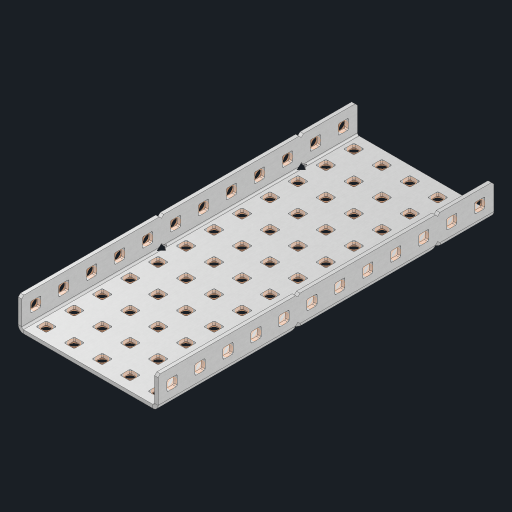
# Autodesk Inventor part: Alu C 1x3x1x35
Saved by Autodesk Inventor 2023 (Build 270158000, 158)
## iProperties
Created: 2022-07-28
Part Number: Alu C 1x3x1x35
Material: Generic
Document SubType Name: Sheet Metal
Designer: ylu12
Density: 1 g/cm^3
Sheet Metal Rule: Default
Appearance: VEX Alu
Author: ylu12
Autodesk Inventor part; units mm, degrees
ref_plane "YZ Plane" through (0, 0, 0) normal (1, 0, 0) x (0, 1, 0)
ref_plane "XZ Plane" through (0, 0, 0) normal (0, 1, 0) x (-1, 0, 0)
sketch "Sketch1" plane through (0, 0, 0) normal (0, 1, 0) x (-1, 0, 0)
  line L0 (-31.75, 0) -> (31.75, 0)
  line L1 (31.75, 0) -> (31.75, -152.4)
  line L2 (31.75, -152.4) -> (-31.75, -152.4)
  line L3 (-31.75, -152.4) -> (-31.75, 0)
  line L4 (31.75, 0) -> (-31.75, -152.4) construction
  point P0 (0, 0)
  point P1 (0, 0)
  dimension "d0" = 63.5
  dimension "d1" = 152.4
  measures "d0" distance of L1.end L2.end
  measures "d1" distance of L0.end L1.end
extrude "Plate1" add sketch "Sketch1" along normal blind 1.5875
sketch "Sketch2" plane through (30.1625, 0, -152.4) normal (1, 0, 0) x (0, 1, 0)
  line L0 (0, 152.4) -> (0, 0)
  line L1 (0, 0) -> (14.2875, 0)
  line L2 (14.2875, 0) -> (14.2875, 152.4)
  line L3 (14.2875, 152.4) -> (0, 152.4)
  constraints: 6 end point, 1 horizontal, 1 perpendicular, 1 vertical
edge flange "Flanges" height 12.7 angle 90 thickness 1.5875 bend radius 0.7937 thickness toward (1, 0, 0) relief tear relief width 1.5875 relief depth 0.7937 corner gap 1.5875 corner form 0 edges at (31.75, 1.5875, -76.2) (-31.75, 1.5875, -76.2) wall of the first edge with corners at (30.1625, 0, 0) (30.1625, 0, -152.4) (30.1625, 14.2875, -152.4) (30.1625, 14.2875, 0)
bend "Bend1"
corner "Corner1"
sketch "Sketch3" plane through (31.75, 2.3813, -152.4) normal (1, 0, 0) x (0, 0, -1)
  line L0 (-147.8534, 7.8676) -> (-144.2466, 7.8676)
  line L1 (-143.7386, 7.3597) -> (-143.7386, 3.7528)
  line L2 (-144.2466, 3.2448) -> (-147.8534, 3.2448)
  line L3 (-148.3614, 3.7528) -> (-148.3614, 7.3597)
  arc A0 (-147.8534, 7.8676) -> (-148.3614, 7.3597) centre (-147.8534, 7.3596) ccw
  arc A1 (-143.7386, 7.3597) -> (-144.2466, 7.8676) centre (-144.2466, 7.3596) ccw
  arc A2 (-144.2466, 3.2448) -> (-143.7386, 3.7528) centre (-144.2466, 3.7528) ccw
  arc A3 (-148.3614, 3.7528) -> (-147.8534, 3.2448) centre (-147.8534, 3.7528) ccw
  line L4 (-152.4, 0) -> (-152.4, 11.9062) construction
  line L5 (-152.4, 11.9062) -> (0, 11.9062) construction
  line L6 (-147.8534, 7.3596) -> (-144.2466, 3.7528) construction
  point P0 (-152.4, -2.3813)
  point P1 (-143.7386, 3.2448)
  point P2 (-148.3614, 3.2448)
  point P3 (-146.05, 5.5562)
  dimension "d16" = 4.6228
  dimension "d17" = 0.508
  dimension "d20" = 6.35
  dimension "d21" = 6.35
  constraints: 10 end point, 8 point on circle, 8 tangent, 4 centre point, 4 point on line, 3 equal radius, 2 parallel, 2 perpendicular, 1 horizontal, 1 midpoint
  measures "d16" distance of point (-143.739, 3.245) point (-148.361, 3.245)
  measures "d17" radius of A0
  measures "d20" distance from line of point (-146.05, 5.556) L4
  measures "d21" distance from line of L5 point (-146.05, 5.556)
extrude "Flange Stamp" cut sketch "Sketch3" against normal blind 1.5875
sketch "Sketch7" plane through (31.75, 2.3813, 0) normal (1, 0, 0) x (0, 0, -1)
  arc A0 (4.5466, 7.8677) -> (4.0386, 7.3597) centre (4.5466, 7.3597) ccw construction
  arc A1 (8.1534, 3.2449) -> (8.6614, 3.7529) centre (8.1534, 3.7529) ccw construction
  circle A2 centre (6.35, 5.5563) radius 2.1844
  line L0 (4.5466, 7.3597) -> (8.1534, 3.7529) construction
  point P0 (0, -2.3812)
  dimension "d46" = 4.3688
  constraints: 2 end point, 1 centre point, 1 midpoint
  measures "d46" diameter of A2
surface extrude "Flange Circle" sketch "Sketch7" against normal up to surface (1.5875 mm away) shown yes curves A2
ref_plane "Flange Pattern Plane" through (31.75, 7.9375, -4.5466) normal (0, 1, 0) x (1, 0, 0)
pattern_sketch "Flange Pattern" of "Flange Circle", "Flange Stamp" from (31.75, 7.9375, -6.35) facing (1, 0, 0) copies at (31.75, 7.9375, -19.05) facing (1, 0, 0) at (31.75, 7.9375, -31.75) facing (1, 0, 0) at (31.75, 7.9375, -44.45) facing (1, 0, 0) at (31.75, 7.9375, -57.15) facing (1, 0, 0) at (31.75, 7.9375, -69.85) facing (1, 0, 0) at (31.75, 7.9375, -82.55) facing (1, 0, 0) at (31.75, 7.9375, -95.25) facing (1, 0, 0) at (31.75, 7.9375, -107.95) facing (1, 0, 0) at (31.75, 7.9375, -120.65) facing (1, 0, 0) at (31.75, 7.9375, -133.35) facing (1, 0, 0) at (31.75, 7.9375, -146.05) facing (1, 0, 0) at (-31.75, 7.9375, -6.35) facing (-1, 0, 0) at (-31.75, 7.9375, -19.05) facing (-1, 0, 0) at (-31.75, 7.9375, -31.75) facing (-1, 0, 0) at (-31.75, 7.9375, -44.45) facing (-1, 0, 0) at (-31.75, 7.9375, -57.15) facing (-1, 0, 0) at (-31.75, 7.9375, -69.85) facing (-1, 0, 0) at (-31.75, 7.9375, -82.55) facing (-1, 0, 0) at (-31.75, 7.9375, -95.25) facing (-1, 0, 0) at (-31.75, 7.9375, -107.95) facing (-1, 0, 0) at (-31.75, 7.9375, -120.65) facing (-1, 0, 0) at (-31.75, 7.9375, -133.35) facing (-1, 0, 0) at (-31.75, 7.9375, -146.05) facing (-1, 0, 0)
sketch "Sketch8" plane through (0, 0, 0) normal (0, -1, 0) x (1, 0, 0)
  line L0 (29.3687, 0) -> (-29.3687, 0) construction
  line L1 (27.2034, -4.0386) -> (23.5966, -4.0386)
  line L2 (23.0886, -4.5466) -> (23.0886, -8.1534)
  line L3 (23.5966, -8.6614) -> (27.2034, -8.6614)
  line L4 (27.7114, -8.1534) -> (27.7114, -4.5466)
  arc A0 (27.7114, -4.5466) -> (27.2034, -4.0386) centre (27.2034, -4.5466) ccw
  arc A1 (27.2034, -8.6614) -> (27.7114, -8.1534) centre (27.2034, -8.1534) ccw
  arc A2 (23.0886, -8.1534) -> (23.5966, -8.6614) centre (23.5966, -8.1534) ccw
  arc A3 (23.5966, -4.0386) -> (23.0886, -4.5466) centre (23.5966, -4.5466) ccw
  line L5 (27.2034, -4.5466) -> (23.5966, -8.1534) construction
  line L6 (31.75, 0) -> (31.75, -152.4) construction
  point P0 (0, 0)
  point P1 (23.0886, -8.6614)
  point P2 (27.7114, -8.6614)
  point P3 (25.4, -6.35)
  dimension "d49" = 4.6228
  dimension "d50" = 0.508
  dimension "d51" = 6.35
  dimension "d52" = 6.35
  constraints: 10 end point, 8 point on circle, 8 tangent, 4 centre point, 4 point on line, 3 equal radius, 2 parallel, 2 perpendicular, 1 horizontal, 1 midpoint
  measures "d49" distance of point (27.711, -8.661) point (23.089, -8.661)
  measures "d50" radius of A0
  measures "d51" distance from line of L6 point (25.4, -6.35)
  measures "d52" distance from line of L0 point (25.4, -6.35)
extrude "Body Stamp" cut sketch "Sketch8" against normal blind 1.5875
sketch "Sketch9" plane through (0, 0, 0) normal (0, -1, 0) x (1, 0, 0)
  arc A0 (27.7114, -4.5466) -> (27.2034, -4.0386) centre (27.2034, -4.5466) ccw construction
  arc A1 (23.0886, -8.1534) -> (23.5966, -8.6614) centre (23.5966, -8.1534) ccw construction
  line L0 (27.2034, -4.5466) -> (23.5966, -8.1534) construction
  circle A2 centre (25.4, -6.35) radius 2.1844
  point P0 (0, 0)
  dimension "d55" = 4.3688
  constraints: 2 end point, 1 centre point, 1 midpoint
  measures "d55" diameter of A2
surface extrude "Body Circle" sketch "Sketch9" against normal up to surface (1.5875 mm away) shown yes curves A2
pattern_sketch "Body Pattern" of "Body Stamp", "Body Circle" from (25.4, 0, -6.35) copies at (25.4, 0, -19.05) at (25.4, 0, -31.75) at (25.4, 0, -44.45) at (25.4, 0, -57.15) at (25.4, 0, -69.85) at (25.4, 0, -82.55) at (25.4, 0, -95.25) at (25.4, 0, -107.95) at (25.4, 0, -120.65) at (25.4, 0, -133.35) at (25.4, 0, -146.05) at (12.7, 0, -6.35) at (12.7, 0, -19.05) at (12.7, 0, -31.75) at (12.7, 0, -44.45) at (12.7, 0, -57.15) at (12.7, 0, -69.85) at (12.7, 0, -82.55) at (12.7, 0, -95.25) at (12.7, 0, -107.95) at (12.7, 0, -120.65) at (12.7, 0, -133.35) at (12.7, 0, -146.05) at (0, 0, -6.35) at (0, 0, -19.05) at (0, 0, -31.75) at (0, 0, -44.45) at (0, 0, -57.15) at (0, 0, -69.85) at (0, 0, -82.55) at (0, 0, -95.25) at (0, 0, -107.95) at (0, 0, -120.65) at (0, 0, -133.35) at (0, 0, -146.05) at (-12.7, 0, -6.35) at (-12.7, 0, -19.05) at (-12.7, 0, -31.75) at (-12.7, 0, -44.45) at (-12.7, 0, -57.15) at (-12.7, 0, -69.85) at (-12.7, 0, -82.55) at (-12.7, 0, -95.25) at (-12.7, 0, -107.95) at (-12.7, 0, -120.65) at (-12.7, 0, -133.35) at (-12.7, 0, -146.05) at (-25.4, 0, -6.35) at (-25.4, 0, -19.05) at (-25.4, 0, -31.75) at (-25.4, 0, -44.45) at (-25.4, 0, -57.15) at (-25.4, 0, -69.85) at (-25.4, 0, -82.55) at (-25.4, 0, -95.25) at (-25.4, 0, -107.95) at (-25.4, 0, -120.65) at (-25.4, 0, -133.35) at (-25.4, 0, -146.05)
sketch "Arc Length" plane through (30.1625, 2.3812, 0) normal (0, 0, 1) x (1, 0, 0)
  line L0 (0, 0) -> (1.5875, 0) construction
  arc A0 (-0.7938, -0.7937) -> (0, 0) centre (-0.7937, 0) ccw construction
  line L1 (-0.7938, -2.3812) -> (-0.7938, -0.7937) construction
  arc A1 (-0.7938, -2.3812) -> (1.5875, 0) centre (-0.7937, 0) ccw construction
  point P0 (-30.1625, -2.3812)
  dimension "d85" = 3.7405
  dimension "d92" = 1.2468
sketch "Sketch13" plane through (31.75, 14.2875, 0) normal (1, 0, 0) x (0, 0, -1)
  line L0 (0, 0) -> (152.4, 0) construction
  line L1 (62.4078, 0) -> (63.4238, -1.016)
  line L2 (63.4238, -1.016) -> (64.4398, 0)
  line L3 (62.4078, 0) -> (64.4398, 0)
  line L4 (152.4, -11.9062) -> (0, -11.9063) construction
  line L5 (63.4238, -10.8903) -> (61.161, -13.1531)
  line L6 (61.161, -13.1531) -> (63.4238, -15.4159)
  line L7 (63.4238, -15.4159) -> (65.6866, -13.1531)
  line L8 (65.6866, -13.1531) -> (63.4238, -10.8903)
  line L9 (63.4238, -10.8903) -> (63.4238, -15.4159) construction
  line L10 (63.4238, -1.016) -> (63.4238, -10.8903) construction
  line L11 (0, -11.9063) -> (152.4, -11.9062) construction
  point P0 (0, -14.2875)
  dimension "d86" = 4.5256
  dimension "d88" = 1.016
  dimension "d91" = 1.016
  dimension "d102" = 63.4238
  constraints: 19 end point, 6 perpendicular, 2 point on line, 2 vertical, 1 collinear
  measures "d86" distance of L5.start L6.end
  measures "d88" distance from line of L0 L1.end
  measures "d91" distance from line of L5.start L11
  measures "d102" distance from line of L0.start L10
cut across bends "Notch" sketch "Sketch13" k factor 0.44
mirror "Notch Mirror" about plane through (0, 0, 0) normal (1, 0, 0) of "Notch"
pattern_linear "Notch Pattern" count 2 spacing 63.5 along (0, 0, -1) of "Notch", "Notch Mirror"
chamfer "End Chamfer" distance 1.016 angle 45 4 edges at (-30.9562, 14.2875, -152.4) (30.9563, 14.2875, -152.4) (-30.9562, 14.2875, 0) (30.9562, 14.2875, 0)
sketch "Sketch14" plane through (-31.75, 2.3812, 292.1) normal (1, 0, 0) x (0, 0, -1)
  line L0 (292.1, 11.9063) -> (444.5, 11.9063) construction
  line L1 (292.1, 0) -> (292.1, 11.9063) construction
  line L2 (292.1, -2.3813) -> (444.5, -2.3812) construction
  line L3 (292.1, 11.9063) -> (444.5, 11.9063)
  line L4 (444.5, 11.9063) -> (444.5, -2.3812)
  line L5 (444.5, -2.3812) -> (292.1, -2.3813)
  line L6 (292.1, -2.3813) -> (292.1, 11.9063)
  point P0 (292.1, -2.3812)
  point P1 (382.0521, -1.9844)
  constraints: 8 end point, 2 collinear, 2 parallel, 1 horizontal, 1 perpendicular, 1 other
extrude "Half Cut" [suppressed]
sketch "Flange Pattern Sketch" plane through (31.75, 7.9375, -4.5466) normal (0, 1, 0) x (1, 0, 0)
  line L0 (0, 3.6068) -> (0, 0) construction
  line L1 (-76.2986, -4.5466) -> (13.2918, -4.5466) construction
  line L2 (0, 0) -> (-1.5875, 0) construction
  point P0 (-31.75, -4.5466)
  point P1 (0, 1.8034)
  point P2 (0, 14.5034)
  point P3 (0, 27.2034)
  point P4 (0, 39.9034)
  point P5 (0, 52.6034)
  point P6 (0, 65.3034)
  point P7 (0, 78.0034)
  point P8 (0, 90.7034)
  point P9 (0, 103.4034)
  point P10 (0, 116.1034)
  point P11 (0, 128.8034)
  point P12 (0, 141.5034)
  point P13 (-63.5, 1.8034)
  point P14 (-63.5, 14.5034)
  point P15 (-63.5, 27.2034)
  point P16 (-63.5, 39.9034)
  point P17 (-63.5, 52.6034)
  point P18 (-63.5, 65.3034)
  point P19 (-63.5, 78.0034)
  point P20 (-63.5, 90.7034)
  point P21 (-63.5, 103.4034)
  point P22 (-63.5, 116.1034)
  point P23 (-63.5, 128.8034)
  point P24 (-63.5, 141.5034)
  dimension "d131" = 63.5
  dimension "d134" = 12.7
  constraints: 1 horizontal, 1 midpoint, 1 vertical, 23 other
  measures "d134" distance of point (0, 1.803) point (0, 14.503)
sketch "Body Pattern Sketch" plane through (0, 0, 0) normal (0, -1, 0) x (1, 0, 0)
  line L0 (29.3687, 0) -> (-29.3687, 0) construction
  line L1 (31.75, 0) -> (31.75, -152.4) construction
  circle A0 centre (25.4, -6.35) radius 2.1844 construction
  point P0 (0, 0)
  point P1 (25.4, -19.05)
  point P2 (25.4, -31.75)
  point P3 (25.4, -44.45)
  point P4 (25.4, -57.15)
  point P5 (25.4, -69.85)
  point P6 (25.4, -82.55)
  point P7 (25.4, -95.25)
  point P8 (25.4, -107.95)
  point P9 (25.4, -120.65)
  point P10 (25.4, -133.35)
  point P11 (25.4, -146.05)
  point P12 (12.7, -6.35)
  point P13 (12.7, -19.05)
  point P14 (12.7, -31.75)
  point P15 (12.7, -44.45)
  point P16 (12.7, -57.15)
  point P17 (12.7, -69.85)
  point P18 (12.7, -82.55)
  point P19 (12.7, -95.25)
  point P20 (12.7, -107.95)
  point P21 (12.7, -120.65)
  point P22 (12.7, -133.35)
  point P23 (12.7, -146.05)
  point P24 (0, -6.35)
  point P25 (0, -19.05)
  point P26 (0, -31.75)
  point P27 (0, -44.45)
  point P28 (0, -57.15)
  point P29 (0, -69.85)
  point P30 (0, -82.55)
  point P31 (0, -95.25)
  point P32 (0, -107.95)
  point P33 (0, -120.65)
  point P34 (0, -133.35)
  point P35 (0, -146.05)
  point P36 (-12.7, -6.35)
  point P37 (-12.7, -19.05)
  point P38 (-12.7, -31.75)
  point P39 (-12.7, -44.45)
  point P40 (-12.7, -57.15)
  point P41 (-12.7, -69.85)
  point P42 (-12.7, -82.55)
  point P43 (-12.7, -95.25)
  point P44 (-12.7, -107.95)
  point P45 (-12.7, -120.65)
  point P46 (-12.7, -133.35)
  point P47 (-12.7, -146.05)
  point P48 (-25.4, -6.35)
  point P49 (-25.4, -19.05)
  point P50 (-25.4, -31.75)
  point P51 (-25.4, -44.45)
  point P52 (-25.4, -57.15)
  point P53 (-25.4, -69.85)
  point P54 (-25.4, -82.55)
  point P55 (-25.4, -95.25)
  point P56 (-25.4, -107.95)
  point P57 (-25.4, -120.65)
  point P58 (-25.4, -133.35)
  point P59 (-25.4, -146.05)
  dimension "d62" = 12.7
  dimension "d65" = 12.7
  dimension "d139" = 12.7
  constraints: 1 coincident, 1 horizontal, 1 vertical, 59 other
  measures "d139" distance of point (25.4, -19.05) point (25.4, -6.35)
equation "\"d1\" = 12.7 * Length"
equation "\"d18\" = Thickness"
equation "\"d53\" = Thickness"
equation "\"d89\" = Thickness"
equation "\"d2\" = Thickness"
equation "\"d3\" = BendReliefWidth"
equation "\"d4\" = BendReliefDepth"
equation "\"d5\" = MinimumRemnant"
equation "\"d6\" = TransitionRadius"
equation "\"d10\" = CornerReliefSize"
equation "\"d11\" = GapSize"
equation "\"d12\" = JacobiRadiusSize"
equation "\"BendRadius\" = Thickness"
equation "\"BendReliefWidth\" = Thickness"
equation "\"BendReliefDepth\" = 0.5 * Thickness"
equation "\"CornerReliefSize\" = 4 * Thickness"
equation "\"MinimumRemnant\" = 2 * Thickness"
equation "\"TransitionRadius\" = BendRadius"
equation "\"JacobiRadiusSize\" = BendRadius"
equation "\"GapSize\" = Thickness"
equation "\"Length\" = 12"
equation "\"Thickness\" = 1.5875"
body "Solid1"
body "Srf1"
body "Srf2"
body "Srf91"
body "Srf92"
body "Srf856"
body "Srf1310"
body "Srf1311"
body "Srf1312"
body "Srf1376"
body "Srf1377"
body "Srf1728"
body "Srf1755"
body "Srf1878"
body "Srf1879"
body "Srf1880"
body "Srf1881"
body "Srf1882"
body "Srf1883"
body "Srf1884"
body "Srf1885"
body "Srf1886"
body "Srf1887"
body "Srf1888"
body "Srf1889"
body "Srf1890"
body "Srf1891"
body "Srf1892"
body "Srf1893"
body "Srf1894"
body "Srf1895"
body "Srf1942"
body "Srf1943"
body "Srf1944"
body "Srf1945"
body "Srf1946"
body "Srf1947"
body "Srf1948"
body "Srf1949"
body "Srf1950"
body "Srf1951"
body "Srf1952"
body "Srf1953"
body "Srf1954"
body "Srf1955"
body "Srf1956"
body "Srf1957"
body "Srf1958"
body "Srf1959"
body "Srf1960"
body "Srf1961"
body "Srf1962"
body "Srf1963"
body "Srf1964"
body "Srf1965"
body "Srf1966"
body "Srf1967"
body "Srf1968"
body "Srf1969"
body "Srf1970"
body "Srf2146"
body "Srf2147"
body "Srf2148"
body "Srf2149"
body "Srf2150"
body "Srf2151"
body "Srf2152"
body "Srf2153"
body "Srf2154"
body "Srf2155"
body "Srf2156"
body "Srf2157"
body "Srf2158"
body "Srf2159"
body "Srf2160"
body "Srf2161"
body "Srf2162"
body "Srf2163"
body "Srf2164"
body "Srf2165"
body "Srf2166"
body "Srf2167"
body "Srf2168"
body "Srf2169"
body "Srf2170"
